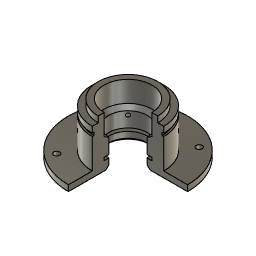
Sketch22_Final v1 (Autodesk Fusion 360 design; units mm, degrees)
Autodesk Fusion 360 part; units mm, degrees
sketch "Sketch1" plane through (0, 0, 0) normal (0, 1, 0) x (1, 0, 0)
  line L0 (-37, 0) -> (-100, 0)
  line L1 (-100, 0) -> (-100, -10)
  line L2 (-100, -10) -> (-60, -10)
  line L3 (0, -10) -> (0, -5)
  line L4 (-32, -5) -> (-37, 0)
  line L5 (-32, -5) -> (-32, -10)
  line L6 (-40, -85) -> (-50, -85)
  line L7 (-40, -85) -> (-40, -50)
  line L8 (-40, -50) -> (-32, -45)
  line L9 (-50, -75) -> (-60, -75)
  line L10 (-50, -85) -> (-50, -75)
  line L11 (-60, -75) -> (-60, -65)
  line L12 (-60, -65) -> (-57, -65)
  line L13 (-57, -65) -> (-57, -60)
  line L14 (-57, -60) -> (-60, -60)
  line L15 (-32, -5) -> (-32, -15)
  line L16 (-32, -15) -> (-40, -15)
  line L17 (-40, -15) -> (-40, -20)
  line L18 (-40, -20) -> (-32, -20)
  line L19 (-60, -10) -> (-60, -60)
  line L20 (-60, -65) -> (-60, -75)
  line L21 (-32, -5) -> (-32, -15)
  line L22 (-32, -20) -> (-32, -45)
  dimension "d1" = 100
  dimension "d2" = 10
  dimension "d5" = 60
  dimension "d15" = 65
  dimension "d16" = 10
  dimension "d17" = 3
  dimension "d19" = 8
  constraint horizontal L0
  constraint perpendicular L0 L1
  constraint perpendicular L1 L2
  constraint perpendicular L0 L3
  constraint perpendicular L2 L5
  constraint perpendicular L0 L21
  constraint perpendicular L6 L21
  constraint perpendicular L9 L19
  constraint perpendicular L9 L10
  constraint perpendicular L9 L11
  constraint perpendicular L12 L19
  constraint perpendicular L12 L13
  constraint perpendicular L14 L19
  constraint perpendicular L14 L15
  constraint perpendicular L16 L21
  constraint perpendicular L16 L17
  constraint coincident L18.end L21
  constraint perpendicular L18 L21
  constraint collinear L19 L20
  constraint collinear L21 L22
  constraint coincident L8.end L21
  measures "d1" distance of origin L0.end
  measures "d2" distance of L0.end L1.end
  measures "d5" distance of L3.start L2.end
  measures "d15" distance of L2.end L9.end
  measures "d16" distance of L9.end L11.end
  measures "d17" distance of L11.end L12.end
  measures "d19" distance of L15.end L16.end
revolve "Revolve1" add sketch "Sketch1" angle 360 about axis through (0, 0, 1.75) along (0, 0, 1) second angle 360
hole "Hole1" at (64.5241, -55.0471, 10) direction (0, 0, -1) diameter 10 depth 10 tip angle 118
pattern_circular "C-Pattern1" count 4 over 360 about axis through (0, 0, 1.75) along (0, 0, 1) of "Hole1"
hole "Hole2" at (-42.4264, -42.4264, 38.7259) direction (0.707107, 0.707107, 0) diameter 6 depth 32 tip angle 118
pattern_circular "C-Pattern2" count 4 over 360 about axis through (0, 0, 1.75) along (0, 0, 1) of "Hole2"
sketch "Sketch2" plane through (0, 0, 0) normal (0, 0, 1) x (1, 0, 0)
  line L0 (0, 0) -> (110, 0)
  line L1 (110, 0) -> (110, -110)
  line L2 (110, -110) -> (0, -110)
  line L3 (0, -110) -> (0, 0)
  constraint horizontal L0
  constraint vertical L1
  constraint horizontal L2
  constraint vertical L3
  constraint coincident L0.start L3.end
extrude "Extrude1" cut sketch "Sketch2" along normal blind 110
